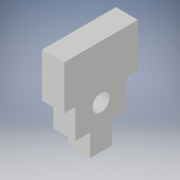
# Autodesk Inventor part: apoio do meioesse
Saved by Autodesk Inventor 2017 (Build 210142000, 142)
## iProperties
Created: 2017-03-09
Part Number: apoio do meioesse
Material: Generic
Document SubType Name: Modeling
Designer: vitor
Density: 1 g/cm^3
Appearance: Default
Author: vitor
Autodesk Inventor part; units mm, degrees
ref_plane "YZ Plane" through (0, 0, 0) normal (1, 0, 0) x (0, 1, 0)
ref_plane "XZ Plane" through (0, 0, 0) normal (0, 1, 0) x (-1, 0, 0)
ref_plane "XY Plane" through (0, 0, 0) normal (0, 0, 1) x (1, 0, 0)
sketch "Sketch1" plane through (0, 0, 0) normal (1, 0, 0) x (0, 1, 0)
  line L0 (2.5746, 9.4872) -> (-17.4254, 9.4872)
  line L1 (-17.4254, 9.4872) -> (-17.4254, -4.5128)
  line L2 (-17.4254, -4.5128) -> (2.5746, -4.5128)
  line L3 (2.5746, -4.5128) -> (2.5746, 9.4872)
  line L4 (2.5746, -4.5128) -> (-9.4254, -4.5128)
  line L5 (-9.4254, -4.5128) -> (-9.4254, -7.5128)
  line L6 (-9.4254, -7.5128) -> (2.5746, -7.5128)
  line L7 (2.5746, -7.5128) -> (2.5746, -4.5128)
  line L8 (2.5746, 9.4872) -> (-9.4254, 9.4872)
  line L9 (-9.4254, 9.4872) -> (-9.4254, 12.4872)
  line L10 (-9.4254, 12.4872) -> (2.5746, 12.4872)
  line L11 (2.5746, 12.4872) -> (2.5746, 9.4872)
  point P0 (0, 0)
  dimension "d0" = 20
  dimension "d1" = 14
  dimension "d2" = 12
  dimension "d3" = 3
  dimension "d4" = 12
  dimension "d5" = 3
  constraints: 24 end point, 6 parallel, 3 horizontal, 3 perpendicular
  measures "d0" distance of L2.end L1.end
  measures "d1" distance of L1.end L0.end
  measures "d2" distance of L6.end L5.end
  measures "d3" distance of L5.end L4.end
  measures "d4" distance of L9.end L10.end
  measures "d5" distance of L8.end L9.end
extrude "Extrusion1" add sketch "Sketch1" along normal blind 6
sketch "Sketch2" plane through (6, 0, 0) normal (1, 0, 0) x (0, 0, -1)
  circle A0 centre (-2.4872, -11.8754) radius 2.3
  line L0 (-9.4872, -17.4254) -> (4.5128, -17.4254) projected
  line L1 (-9.4872, -9.4254) -> (-9.4872, -17.4254) projected
  point P0 (0, 0)
  dimension "d8" = 4.6
  dimension "d9" = 5.55
  dimension "d10" = 7
  constraints: 1 centre point
  measures "d8" diameter of A0
  measures "d9" distance from line of L0 A0.centre
  measures "d10" distance from line of L1 A0.centre
extrude "Extrusion2" cut sketch "Sketch2" against normal blind 6
sketch "Sketch3" plane through (6, 0, 0) normal (1, 0, 0) x (0, 0, -1)
  line L0 (-5.4872, -17.4254) -> (0.5128, -17.4254)
  line L1 (0.5128, -17.4254) -> (0.5128, -23.4254)
  line L2 (0.5128, -23.4254) -> (-5.4872, -23.4254)
  line L3 (-5.4872, -23.4254) -> (-5.4872, -17.4254)
  line L4 (-9.4872, -9.4254) -> (-9.4872, -17.4254) construction
  line L5 (-9.4872, -17.4254) -> (-5.4872, -17.4254) construction
  line L6 (0.5128, -17.4254) -> (4.5128, -17.4254) construction
  line L7 (-9.4872, -17.4254) -> (4.5128, -17.4254) construction
  point P0 (0, 0)
  dimension "d13" = 6
  dimension "d14" = 6
  constraints: 12 end point, 2 collinear, 2 parallel, 1 horizontal, 1 perpendicular
  measures "d13" distance of L1.end L2.end
  measures "d14" distance of L0.end L1.end
extrude "Extrusion3" add sketch "Sketch3" against normal blind 6
body "Solid1"
